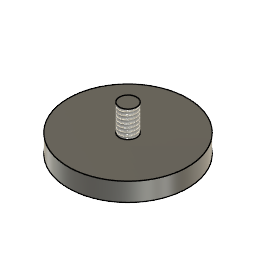
Laser Monitor Assembly (Autodesk Fusion 360 archive; units mm, degrees)
design "Magnet Base"
Autodesk Fusion 360 part; units mm, degrees
sketch "Sketch1" plane through (0, 0, 0) normal (0, 0, 1) x (1, 0, 0)
  circle A0 centre (0, 0) radius 21.463
  dimension "d1" = 42.926
  constraint coincident A0.centre origin
  measures "d1" diameter of A0
extrude "Extrude1" add sketch "Sketch1" along normal blind 5
sketch "Sketch2" plane through (0, 0, 5) normal (0, 0, 1) x (-1, 0, 0)
  circle A0 centre (0, 0) radius 21.463
  circle A1 centre (0, 0) radius 3.175
  dimension "d4" = 6.35
  constraint coincident A0.centre A1.centre
  measures "d4" diameter of A1
extrude "Extrude2" add sketch "Sketch2" along normal blind 9.4996 contours A1
thread "Thread1" "ANSI Unified Screw Threads 0.25 1/4-20 UNC 1/4-20 UNC 3A" major diameter 6.2484 minor diameter 4.8387 pitch 1.27 angle 60 resizes the face on face at (-3.1711, 0.1583, 11.3331)
move_face "OffsetFaces1" offset 1.651 1 faces at (6.8365, 2.1088, 0)
equation "d5 = -0.385 in + 0.709 in + 0.05 in"
equation "d9 = 0.262 in - 0.197 in"

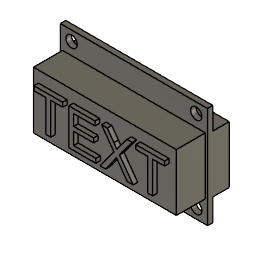
design "14 Segment Module"
Autodesk Fusion 360 part; units mm, degrees
sketch "Sketch1" plane through (0, 0, 0) normal (0, 1, 0) x (1, 0, 0)
  line L0 (0, 0) -> (41.275, 0)
  line L1 (41.275, 0) -> (41.275, -28.448)
  line L2 (41.275, -28.448) -> (0, -28.448)
  line L3 (0, -28.448) -> (0, 0)
  dimension "d1" = 41.275
  dimension "d2" = 28.448
  constraint horizontal L0
  constraint vertical L1
  constraint horizontal L2
  constraint vertical L3
  constraint coincident L0.start L3.end
  measures "d1" distance of L0.start L0.end
  measures "d2" distance of L0.start L2.end
extrude "Extrude1" add sketch "Sketch1" along normal blind 1.524
sketch "Sketch2" plane through (0, 0, 0) normal (0, -1, 0) x (1, 0, 0)
  line L0 (41.275, 28.448) -> (0, 28.448)
  line L1 (0, 28.448) -> (0, 0)
  line L2 (0, 0) -> (41.275, 0)
  line L3 (41.275, 0) -> (41.275, 28.448)
  line L4 (3.175, 25.654) -> (38.1, 25.654) construction
  line L5 (38.1, 25.654) -> (38.1, 2.794) construction
  line L6 (38.1, 2.794) -> (3.175, 2.794) construction
  line L7 (3.175, 2.794) -> (3.175, 25.654) construction
  line L8 (3.175, 25.654) -> (38.1, 2.794) construction
  line L9 (38.1, 25.654) -> (3.175, 2.794) construction
  line L10 (0, 28.448) -> (41.275, 0) construction
  line L11 (41.275, 28.448) -> (0, 0) construction
  circle A0 centre (3.175, 25.654) radius 1.5875
  circle A1 centre (3.175, 2.794) radius 1.5875
  circle A2 centre (38.1, 2.794) radius 1.5875
  circle A3 centre (38.1, 25.654) radius 1.5875
  point P0 (20.6375, 14.224)
  dimension "d5" = 34.925
  dimension "d6" = 22.86
  dimension "d7" = 3.175
  dimension "d8" = 3.175
  dimension "d9" = 3.175
  dimension "d10" = 3.175
  constraint horizontal L4
  constraint perpendicular L4 L5
  constraint parallel L4 L6
  constraint parallel L5 L7
  constraint coincident L8 P0
  constraint coincident L9 P0
  constraint coincident L0.end L1.start
  constraint coincident L2.end L3.start
  constraint coincident L0.start L3.end
  constraint coincident L1.end L2.start
  constraint coincident L4.start L7.end
  constraint coincident L6.end L7.start
  constraint coincident L5.end L6.start
  constraint coincident L4.end L5.start
  measures "d5" distance of L5.end L6.end
  measures "d6" distance of L4.end L5.end
  measures "d7" diameter of A0
  measures "d8" diameter of A1
  measures "d9" diameter of A2
  measures "d10" diameter of A3
extrude "Extrude2" cut sketch "Sketch2" against normal blind 7.62 contours A0 | A1 | A2 | A3
sketch "Sketch3" plane through (0, 0, 0) normal (0, -1, 0) x (1, 0, 0)
  circle A0 centre (3.175, 25.654) radius 1.5875
  circle A1 centre (3.175, 2.794) radius 1.5875
  circle A2 centre (38.1, 25.654) radius 1.5875
  circle A3 centre (38.1, 2.794) radius 1.5875
  line L0 (41.275, 28.448) -> (0, 28.448)
  line L1 (0, 28.448) -> (0, 0)
  line L2 (0, 0) -> (41.275, 0)
  line L3 (41.275, 0) -> (41.275, 28.448)
  line L4 (0, 14.224) -> (41.275, 14.224) construction
  line L5 (0, 22.225) -> (41.275, 22.225)
  line L6 (41.275, 22.225) -> (41.275, 6.223)
  line L7 (41.275, 6.223) -> (0, 6.223)
  line L8 (0, 6.223) -> (0, 22.225)
  line L9 (0, 22.225) -> (41.275, 6.223) construction
  line L10 (41.275, 22.225) -> (0, 6.223) construction
  point P0 (20.6375, 14.224)
  dimension "d13" = 16.002
  constraint midpoint L1 L4.start
  constraint midpoint L3 L4.end
  constraint horizontal L5
  constraint perpendicular L5 L6
  constraint parallel L5 L7
  constraint parallel L6 L8
  constraint coincident L9 P0
  constraint coincident L10 P0
  constraint midpoint L4 P0
  measures "d13" distance of L5.end L6.end
extrude "Extrude3" add sketch "Sketch3" along normal blind 8.128 contours L1 L3 L5 L6 L7 L8
sketch "Sketch4" plane through (0, 1.524, 0) normal (0, 1, 0) x (-1, 0, 0)
  circle A0 centre (-3.175, 25.654) radius 1.5875
  circle A1 centre (-3.175, 2.794) radius 1.5875
  circle A2 centre (-38.1, 25.654) radius 1.5875
  circle A3 centre (-38.1, 2.794) radius 1.5875
  line L0 (0, 28.448) -> (-41.275, 28.448)
  line L1 (-41.275, 28.448) -> (-41.275, 0)
  line L2 (-41.275, 0) -> (0, 0)
  line L3 (0, 0) -> (0, 28.448)
  line L4 (0, 6.223) -> (-41.275, 6.223)
  line L5 (-41.275, 6.223) -> (-41.275, 22.225)
  line L6 (-41.275, 22.225) -> (0, 22.225)
  line L7 (0, 22.225) -> (0, 6.223)
extrude "Extrude4" add sketch "Sketch4" along normal blind 4.572 contours L1 L3 L4 L5 L6 L7
sketch "Sketch5" plane through (0, -8.128, 0) normal (0, -1, 0) x (1, 0, 0)
  line L0 (0, 6.223) -> (41.275, 6.223)
  line L1 (41.275, 6.223) -> (41.275, 22.225)
  line L2 (41.275, 22.225) -> (0, 22.225)
  line L3 (0, 22.225) -> (0, 6.223)
  line L4 (2.54, 7.62) -> (38.1, 7.62) construction
  line L5 (38.1, 7.62) -> (38.1, 20.32) construction
  line L6 (38.1, 20.32) -> (2.54, 20.32) construction
  line L7 (2.54, 20.32) -> (2.54, 7.62) construction
  dimension "d18" = 10.16
  text T0 "TEXT" font "Arial" height 10.16 align centre middle in box 35.56 x 12.7 at (2.54, 7.62) x (1, 0) y (0, 1) spacing 1.05 kerned
extrude "Extrude5" add sketch "Sketch5" along normal blind 1.27 text T0
sketch "Sketch6" plane through (0, -8.128, 0) normal (0, -1, 0) x (1, 0, 0)
  line L0 (5.369, 8.89) -> (5.369, 17.851)
  line L1 (5.369, 17.851) -> (2.0216, 17.851)
  line L2 (2.0216, 17.851) -> (2.0216, 19.05)
  line L3 (2.0216, 19.05) -> (10.0748, 19.05)
  line L4 (10.0748, 19.05) -> (10.0748, 17.851)
  line L5 (10.0748, 17.851) -> (6.7135, 17.851)
  line L6 (6.7135, 17.851) -> (6.7135, 8.89)
  line L7 (6.7135, 8.89) -> (5.369, 8.89)
  line L8 (33.9126, 8.89) -> (33.9126, 17.851)
  line L9 (33.9126, 17.851) -> (30.5652, 17.851)
  line L10 (30.5652, 17.851) -> (30.5652, 19.05)
  line L11 (30.5652, 19.05) -> (38.6184, 19.05)
  line L12 (38.6184, 19.05) -> (38.6184, 17.851)
  line L13 (38.6184, 17.851) -> (35.2571, 17.851)
  line L14 (35.2571, 17.851) -> (35.2571, 8.89)
  line L15 (35.2571, 8.89) -> (33.9126, 8.89)
  line L16 (20.5147, 8.89) -> (24.4443, 14.1848)
  line L17 (24.4443, 14.1848) -> (20.9791, 19.05)
  line L18 (20.9791, 19.05) -> (22.58, 19.05)
  line L19 (22.58, 19.05) -> (24.4235, 16.4442)
  spline S0 degree 3 poles (24.4235, 16.4442) (24.5911, 16.2074) (24.8786, 15.8012) (25.1345, 15.3746) (25.2413, 15.1967) knots 0 0 0 0 0.086985 0.14921 0.14921 0.14921 0.14921
  spline S1 degree 3 poles (25.2413, 15.1967) (25.3625, 15.3872) (25.6149, 15.7838) (25.8981, 16.159) (26.0452, 16.3541) knots 0 0 0 0 0.06771 0.140969 0.140969 0.140969 0.140969
  line L20 (26.0452, 16.3541) -> (28.0897, 19.05)
  line L21 (28.0897, 19.05) -> (29.552, 19.05)
  line L22 (29.552, 19.05) -> (25.9829, 14.2611)
  line L23 (25.9829, 14.2611) -> (29.8292, 8.89)
  line L24 (29.8292, 8.89) -> (28.1659, 8.89)
  line L25 (28.1659, 8.89) -> (25.6086, 12.5146)
  spline S2 degree 3 poles (25.6086, 12.5146) (25.5352, 12.6228) (25.3834, 12.8466) (25.2394, 13.0755) (25.1651, 13.1938) knots 0 0 0 0 0.039212 0.081124 0.081124 0.081124 0.081124
  spline S3 degree 3 poles (25.1651, 13.1938) (25.0693, 13.0371) (24.9121, 12.78) (24.7451, 12.5293) (24.6799, 12.4314) knots 0 0 0 0 0.055097 0.090369 0.090369 0.090369 0.090369
  line L26 (24.6799, 12.4314) -> (22.1295, 8.89)
  line L27 (22.1295, 8.89) -> (20.5147, 8.89)
  line L28 (11.7949, 8.89) -> (11.7949, 19.05)
  line L29 (11.7949, 19.05) -> (19.1411, 19.05)
  line L30 (19.1411, 19.05) -> (19.1411, 17.851)
  line L31 (19.1411, 17.851) -> (13.1394, 17.851)
  line L32 (13.1394, 17.851) -> (13.1394, 14.7393)
  line L33 (13.1394, 14.7393) -> (18.76, 14.7393)
  line L34 (18.76, 14.7393) -> (18.76, 13.5472)
  line L35 (18.76, 13.5472) -> (13.1394, 13.5472)
  line L36 (13.1394, 13.5472) -> (13.1394, 10.089)
  line L37 (13.1394, 10.089) -> (19.3768, 10.089)
  line L38 (19.3768, 10.089) -> (19.3768, 8.89)
  line L39 (19.3768, 8.89) -> (11.7949, 8.89)
  line L40 (0, 6.223) -> (41.275, 6.223)
  line L41 (41.275, 6.223) -> (41.275, 22.225)
  line L42 (41.275, 22.225) -> (0, 22.225)
  line L43 (0, 22.225) -> (0, 6.223)
  line L44 (0, 22.225) -> (41.275, 6.223) construction
  line L45 (41.275, 22.225) -> (0, 6.223) construction
  line L46 (0.6223, 22.225) -> (40.6527, 22.225)
  line L47 (40.6527, 22.225) -> (40.6527, 6.223)
  line L48 (40.6527, 6.223) -> (0.6223, 6.223)
  line L49 (0.6223, 6.223) -> (0.6223, 22.225)
  line L50 (0.6223, 22.225) -> (40.6527, 6.223) construction
  line L51 (40.6527, 22.225) -> (0.6223, 6.223) construction
  point P0 (20.6375, 14.224)
  dimension "d22" = 40.0304
  constraint coincident L42.end L43.start
  constraint coincident L40.end L41.start
  constraint coincident L41.end L42.start
  constraint coincident L40.start L43.end
  constraint horizontal L46
  constraint perpendicular L46 L47
  constraint parallel L46 L48
  constraint parallel L47 L49
  constraint coincident L50 P0
  constraint coincident L51 P0
  constraint midpoint L44 P0
  measures "d22" distance of L47.end L48.end
extrude "Extrude6" cut sketch "Sketch6" against normal up to surface (8.128 mm away) contours L40 L42 L43 L49 | L40 L41 L42 L47
equation "d19 = 'TEXT'"
